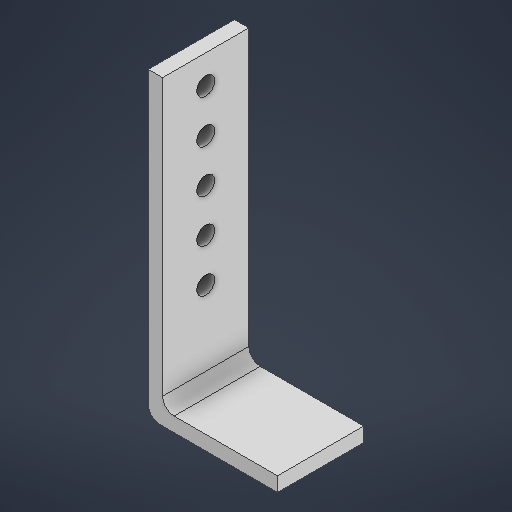
# Autodesk Inventor part: Mounting Bracket
Saved by Autodesk Inventor 2027 (Build 310192000, 192)
## iProperties
Created: 2026-07-15
Part Number: Mounting Bracket
Material: Generic
Document SubType Name: Modeling
Designer: ratik
Density: 1 g/cm^3
Appearance: Default
Author: ratik
Autodesk Inventor part; units mm, degrees
ref_plane "YZ Plane" through (0, 0, 0) normal (1, 0, 0) x (0, 1, 0)
ref_plane "XZ Plane" through (0, 0, 0) normal (0, 1, 0) x (-1, 0, 0)
ref_plane "XY Plane" through (0, 0, 0) normal (0, 0, 1) x (1, 0, 0)
sketch "Sketch1" plane through (0, 0, 0) normal (0, 0, 1) x (1, 0, 0)
  line L0 (-18.2895, 105.4386) -> (-13.2895, 105.4386)
  line L1 (-13.2895, 105.4386) -> (-13.2895, 5.4386)
  line L2 (-18.2895, 84.1228) -> (-18.2895, 105.4386)
  line L3 (-13.2895, 5.4386) -> (26.7105, 5.4386)
  line L4 (26.7105, 5.4386) -> (26.7105, 0.4386)
  line L5 (26.7105, 0.4386) -> (-18.2895, 0.4386)
  line L6 (-18.2895, 0.4386) -> (-18.2895, 84.1228)
  point P0 (0, 0)
  dimension "d0" = 5
  dimension "d1" = 5
  dimension "d2" = 100
  dimension "d3" = 40
  constraints: 14 end point, 3 parallel, 2 horizontal, 2 perpendicular
  measures "d0" distance of L0.start L0.end
  measures "d1" distance of L3.end L4.end
  measures "d2" distance of L0.end L1.end
  measures "d3" distance of L1.end L3.end
extrude "Extrusion1" add sketch "Sketch1" along normal blind 30
fillet "Fillet1" radius 4 2 edges at (-18.2895, 0.4386, 15) (-13.2895, 5.4386, 15)
sketch "Sketch2" plane through (-13.2895, 105.4386, 30) normal (1, 0, 0) x (0, 0, -1)
  circle A0 centre (15, -10) radius 3.1
  line L0 (30, -96) -> (30, 0) projected
  line L1 (30, 0) -> (0, 0) projected
  circle A1 centre (15, -25) radius 3.1
  circle A2 centre (15, -40) radius 3.1
  circle A3 centre (15, -55) radius 3.1
  circle A4 centre (15, -70) radius 3.1
  point P0 (30, -105.4386)
  dimension "d7" = 6.2
  dimension "d8" = 15
  dimension "d9" = 10
  dimension "d13" = 15
  constraints: 5 centre point, 1 vertical, 8 other
  measures "d7" diameter of A0
  measures "d8" distance from line of L0 A0.centre
  measures "d9" distance from line of L1 A0.centre
  measures "d13" distance of A0.centre A1.centre
extrude "Extrusion2" cut sketch "Sketch2" against normal through all
body "Solid1"
